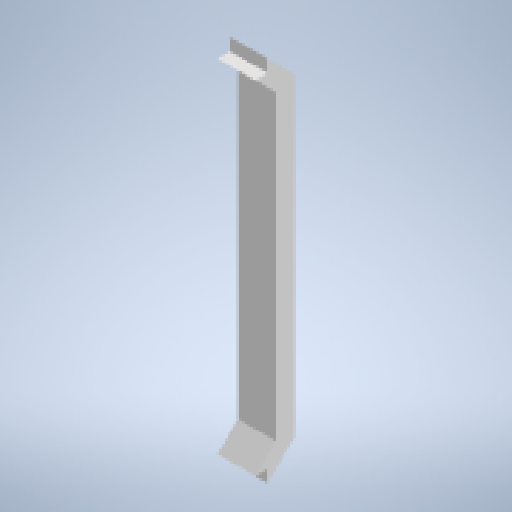
# Autodesk Inventor part: DOF5
Saved by Autodesk Inventor 2024 (Build 280153000, 153)
## iProperties
Created: 2024-10-16
Part Number: DOF5
Material: 一般
Document SubType Name: Modeling
Designer: jerry
Density: 1 g/cm^3
Appearance: 預設
Author: jerry
Autodesk Inventor part; units mm, degrees
ref_plane "YZ Plane" through (0, 0, 0) normal (1, 0, 0) x (0, 1, 0)
ref_plane "XZ Plane" through (0, 0, 0) normal (0, 1, 0) x (-1, 0, 0)
ref_plane "XY Plane" through (0, 0, 0) normal (0, 0, 1) x (1, 0, 0)
sketch "草圖1" plane through (0, 0, 0) normal (0, 0, 1) x (1, 0, 0)
  line L0 (30, -250) -> (-30, -250)
  line L1 (-30, -250) -> (-30, 250)
  line L2 (-30, 250) -> (30, 250)
  line L3 (30, 250) -> (30, -250)
  line L4 (30, -250) -> (-30, 250) construction
  line L5 (-30, -250) -> (30, 250) construction
  point P0 (0, 0)
  dimension "d0" = 60
  dimension "d1" = 500
  constraints: 12 end point, 2 midpoint, 2 parallel, 1 horizontal, 1 perpendicular
  measures "d0" distance of L1.end L2.end
  measures "d1" distance of L0.end L1.end
extrude "擠出1" add sketch "草圖1" along normal blind 30
sketch "草圖2" plane through (30, -250, 0) normal (1, 0, 0) x (0, 0, -1)
  line L0 (0, 500) -> (0, 0) projected
  line L1 (0, 0) -> (-42.4264, -42.4264)
  line L2 (0, 0) -> (60, 0) construction
  line L3 (-42.4264, -42.4264) -> (-42.4264, -22.4264)
  line L4 (-42.4264, -22.4264) -> (-62.4264, -22.4264)
  line L5 (-62.4264, -22.4264) -> (-23.4773, 16.5227)
  line L6 (0, 0) -> (-23.4773, 16.5227)
  line L7 (0, 500) -> (-42.4264, 542.4264)
  line L8 (-42.4264, 542.4264) -> (-42.4264, 522.4264)
  line L9 (-42.4264, 522.4264) -> (-62.4264, 522.4264)
  line L10 (-62.4264, 522.4264) -> (-16.5227, 476.5227)
  line L11 (-16.5227, 476.5227) -> (0, 500)
  point P0 (0, 250)
  dimension "d4" = 60
  dimension "d5" = 135
  dimension "d6" = 20
  dimension "d7" = 20
  dimension "d8" = 60
  dimension "d9" = 20
  dimension "d10" = 20
  constraints: 22 end point, 4 perpendicular, 2 vertical, 1 equal length, 1 horizontal, 1 parallel
  measures "d4" distance of L0.end L1.end
  measures "d5" angle of L1 L2
  measures "d6" distance of L1.end L3.end
  measures "d7" distance of L3.end L4.end
  measures "d8" distance of L0.start L7.end
  measures "d9" distance of L7.end L8.end
  measures "d10" distance of L8.end L9.end
extrude "擠出2" add sketch "草圖2" against normal blind 60
